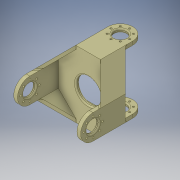
# Autodesk Inventor part: Coaxa 3 Machining
Saved by Autodesk Inventor 2016 (Build 200138000, 138)
## iProperties
Created: 2016-05-19
Part Number: Coaxa 3 Machining
Material: PET Plastic
Document SubType Name: Modeling
Designer: kromm.je.s
Density: 1.541 g/cm^3
Appearance: Smooth - Ash
Mass: 22.5167 g
Surface Area: 110.836 cm^2
Volume: 14.6118 cm^3
Author: kromm.je.s
Autodesk Inventor part; units mm, degrees
ref_plane "YZ Plane" through (0, 0, 0) normal (1, 0, 0) x (0, 1, 0)
sketch "Sketch1" plane through (0, 0, 0) normal (0, 0, 1) x (1, 0, 0)
  circle A0 centre (0, 0) radius 5
  circle A1 centre (0, 0) radius 10
  line L0 (0, 0) -> (-23, 0)
  line L1 (-23, 0) -> (-23, 27)
  line L2 (-23, 0) -> (-23, -27)
  line L3 (0, -10) -> (-23, -10)
  line L4 (0, 10) -> (-23, 10)
  line L5 (-23, 27) -> (-26, 27)
  line L6 (-26, 27) -> (-26, -27)
  line L7 (-26, -27) -> (-23, -27)
  dimension "d0" = 10
  dimension "d1" = 20
  dimension "d2" = 23
  dimension "d3" = 27
  dimension "d4" = 27
  dimension "d5" = 3
  constraints: 16 end point, 4 perpendicular, 3 point on line, 2 centre point, 2 coincident, 2 point on circle, 1 horizontal, 1 parallel, 1 tangent, 1 vertical
  measures "d0" diameter of A0
  measures "d1" diameter of A1
  measures "d2" distance of L0.start L0.end
  measures "d3" distance of L0.end L1.end
  measures "d4" distance of L0.end L2.end
  measures "d5" distance of L1.end L5.end
extrude "Extrusion1" add sketch "Sketch1" along normal blind 54
sketch "Sketch2" plane through (-23, 10, 0) normal (0, 1, 0) x (1, 0, 0)
  line L0 (0, 0) -> (-3, 0) projected
  line L1 (-3, 0) -> (-3, -54) projected
  line L2 (0, -54) -> (-3, -54) projected
  line L3 (0, 0) -> (0, -54) projected
  line L4 (23, 0) -> (0, 0) projected
  line L5 (0, -54) -> (0, 0) projected
  line L6 (23, -54) -> (0, -54) projected
  line L7 (23, 0) -> (23, -54) projected
  line L8 (23, 0) -> (23, -54) projected
  line L9 (23, -54) -> (23, -54) projected
  line L10 (23, 0) -> (23, -54) projected
  line L11 (23, 0) -> (23, 0) projected
  line L12 (0, 0) -> (23, 0) projected
  line L13 (0, 0) -> (0, -3)
  line L14 (0, -54) -> (0, -51)
  line L15 (0, 0) -> (0, -54) projected
  line L16 (33, 0) -> (33, -54) projected
  line L17 (0, -51) -> (33, -51)
  line L18 (33, -51) -> (33, -3)
  line L19 (33, -3) -> (0, -3)
  line L20 (0, -3) -> (0, -51)
  dimension "d8" = 3
  dimension "d9" = 3
  constraints: 12 end point, 3 point on line, 2 parallel, 1 horizontal, 1 perpendicular
  measures "d8" distance of L0.start L13.end
  measures "d9" distance of L5.start L14.end
extrude "Extrusion2" cut sketch "Sketch2" against normal blind 48 contours L19 L7 L17 L3 | L19 L16 L17 L7
sketch "Sketch3" plane through (-26, 27, 0) normal (0, 1, 0) x (1, 0, 0)
  line L0 (3, 0) -> (0, 0) projected
  line L1 (0, 0) -> (0, -54) projected
  line L2 (3, -54) -> (0, -54) projected
  line L3 (3, 0) -> (3, -54) projected
  line L4 (0, 0) -> (0, -54) projected
  line L5 (0, -27) -> (-23, -27)
  circle A0 centre (-23, -27) radius 5
  circle A1 centre (-23, -27) radius 10
  line L6 (-23, -17) -> (0, -17)
  line L7 (-23, -37) -> (0, -37)
  point P0 (26, 0)
  dimension "d12" = 23
  dimension "d13" = 10
  dimension "d14" = 20
  constraints: 6 end point, 2 centre point, 2 coincident, 2 perpendicular, 2 point on circle, 2 point on line, 1 horizontal, 1 midpoint, 1 tangent
  measures "d12" distance of L5.start L5.end
  measures "d13" diameter of A0
  measures "d14" diameter of A1
extrude "Extrusion3" add sketch "Sketch3" against normal blind 54 contours L1 L5 A1 L6 | L1 L7 A1 L5 | A1
sketch "Sketch4" plane through (0, 0, 0) normal (0, 0, -1) x (-1, 0, 0)
  line L0 (26, 27) -> (49, 27) projected
  line L1 (26, -27) -> (26, 27) projected
  line L2 (49, -27) -> (26, -27) projected
  line L3 (49, 27) -> (49, -27) projected
  line L4 (26, 27) -> (26, 24)
  line L5 (26, -27) -> (26, -24)
  line L6 (26, -27) -> (26, 27) projected
  line L7 (59, 27) -> (59, -27) projected
  line L8 (26, 21) -> (26, -24)
  line L9 (26, 24) -> (59, 24)
  line L10 (59, 24) -> (59, -24)
  line L11 (59, -24) -> (26, -24)
  line L12 (26, -24) -> (26, 24)
  point P0 (0, 0)
  dimension "d17" = 3
  dimension "d18" = 3
  constraints: 14 end point, 3 point on line, 2 parallel, 1 horizontal, 1 perpendicular
  measures "d17" distance of L0.start L4.end
  measures "d18" distance of L1.start L5.end
extrude "Extrusion4" cut sketch "Sketch4" against normal blind 48 contours L9 L3 L11 L1 | L9 L7 L11 L3
sketch "Sketch5" plane through (-26, -27, 54) normal (-1, 0, 0) x (0, 0, 1)
  line L0 (0, 54) -> (0, 0) projected
  line L1 (-17, 54) -> (0, 54) projected
  line L2 (-17, 3) -> (-17, 0) projected
  line L3 (-37, 51) -> (-37, 54) projected
  line L4 (-54, 54) -> (-37, 54) projected
  line L5 (-54, 54) -> (-54, 0) projected
  line L6 (-54, 0) -> (-37, 0) projected
  line L7 (-3, 17) -> (0, 17) projected
  line L8 (-3, 17) -> (0, 17) projected
  line L9 (0, 37) -> (-3, 37) projected
  line L10 (-3, 37) -> (0, 37) projected
  line L11 (-54, 37) -> (-51, 37) projected
  line L12 (-51, 37) -> (-54, 37) projected
  line L13 (-54, 17) -> (-51, 17) projected
  line L14 (-54, 17) -> (-51, 17) projected
  line L15 (-54, 17) -> (-51, 17) projected
  line L16 (-37, 0) -> (-54, 17)
  line L17 (-54, 54) -> (-37, 54) projected
  line L18 (-54, 37) -> (-37, 54)
  line L19 (0, 37) -> (-17, 54)
  line L20 (-17, 0) -> (0, 0) projected
  line L21 (-17, 0) -> (0, 17)
  line L22 (0, 0) -> (0, 17) projected
  line L23 (0, 54) -> (0, 0) projected
  line L24 (0, 17) -> (0, 0)
  line L25 (-17, 3) -> (-17, 0) projected
  line L26 (0, 0) -> (-17, 0)
  line L27 (-54, 0) -> (-37, 0) projected
  line L28 (-37, 0) -> (-54, 0)
  line L29 (-54, 0) -> (-54, 17) projected
  line L30 (-54, 0) -> (-54, 17)
  line L31 (-54, 37) -> (-54, 54)
  line L32 (-54, 54) -> (-37, 54)
  line L33 (0, 40) -> (0, 54)
  line L34 (0, 54) -> (-17, 54)
  line L35 (-54, 54) -> (0, 54) projected
  line L36 (-17, 0) -> (0, 0) projected
  line L37 (-37, 0) -> (-37, 3) projected
  line L38 (-37, 3) -> (-17, 3) projected
  line L39 (-17, 54) -> (-17, 51) projected
  line L40 (-37, 51) -> (-17, 51) projected
  point P0 (-54, 27)
  constraints: 24 end point, 4 collinear, 2 vertical, 1 horizontal, 1 perpendicular
extrude "Extrusion5" cut sketch "Sketch5" against normal blind 48 contours L0 L19 L1 | L18 L5 L4 | L0 L20 L21 | L16 L6 L5
sketch "Sketch6" plane through (-23, 27, 37) normal (1, 0, 0) x (0, 0, -1)
  line L0 (37, -17) -> (20, 0) projected
  line L1 (20, 0) -> (0, 0) projected
  line L2 (0, 0) -> (-17, -17) projected
  line L3 (-14, -17) -> (-14, -37) projected
  line L4 (-17, -37) -> (0, -54) projected
  line L5 (20, -54) -> (0, -54) projected
  line L6 (20, -54) -> (37, -37) projected
  line L7 (34, -17) -> (34, -37) projected
  line L8 (20, 0) -> (0, 0) projected
  line L9 (10, 0) -> (10, -54)
  circle A0 centre (10, -27) radius 10
  line L10 (-17, -17) -> (-14, -17) projected
  line L11 (-14, -37) -> (-17, -37) projected
  line L12 (37, -37) -> (34, -37) projected
  line L13 (34, -17) -> (37, -17) projected
  point P0 (37, -27)
  dimension "d26" = 20
  constraints: 3 midpoint, 2 end point, 1 centre point
  measures "d26" diameter of A0
extrude "Extrusion6" cut sketch "Sketch6" against normal blind 48 contours A0 L9 | L9 A0
sketch "Sketch7" plane through (-49, -27, 27) normal (0, -1, 0) x (1, 0, 0)
  circle A0 centre (0, 0) radius 7.5
  circle A1 centre (-7.5, 0) radius 0.75
  point P0 (49, -27)
  dimension "d32" = 15
  dimension "d33" = 1.5
  constraints: 1 centre point, 1 horizontal alignment, 2 other
  measures "d33" diameter of A1
extrude "Extrusion7" cut sketch "Sketch7" against normal blind 56 contours A1 A0 | A0 A1 picked at (-7.2472, 0) picked at (-7.7453, 0.0311)
pattern_circular "Circular Pattern1" count 8 over 360 about axis through (-49, 27, 27) along (0, -1, 0) of "Extrusion7"
sketch "Sketch8" plane through (0, 0, 0) normal (0, 0, -1) x (-1, 0, 0)
  circle A0 centre (0, 0) radius 7.5
  circle A1 centre (-7.5, 0) radius 0.75
  dimension "d39" = 15
  dimension "d40" = 1.5
  constraints: 1 centre point, 1 coincident, 1 horizontal alignment, 2 other
  measures "d40" diameter of A1
extrude "Extrusion8" cut sketch "Sketch8" against normal blind 56 contours A1 A0 | A0 A1 picked at (-7.2472, 0) picked at (-7.7453, 0.0311)
pattern_circular "Circular Pattern2" count 8 over 360 about axis through (0, 0, 0) along (0, 0, 1) of "Extrusion8"
chamfer "Chamfer3" [suppressed]
chamfer "Chamfer4" [suppressed]
sketch "Sketch9" plane through (-26, -10, 0) normal (-1, 0, 0) x (0, 0, 1)
  circle A0 centre (27, 10) radius 10 projected
  line L0 (0, 20) -> (17, 37) projected
  line L1 (17, 37) -> (37, 37) projected
  line L2 (37, 37) -> (54, 20) projected
  line L3 (54, 0) -> (37, -17) projected
  line L4 (17, -17) -> (37, -17) projected
  line L5 (17, -17) -> (0, 0) projected
  line L6 (54, 0) -> (37, -17) projected
  line L7 (37, -17) -> (37, -14)
  line L8 (37, -14) -> (40, -14)
  line L9 (37, -17) -> (40, -14)
  line L10 (17, -17) -> (17, -14)
  line L11 (17, -14) -> (14, -14)
  line L12 (14, -14) -> (17, -17)
  line L13 (0, 20) -> (17, 37) projected
  line L14 (17, 37) -> (17, 34)
  line L15 (17, 34) -> (14, 34)
  line L16 (14, 34) -> (17, 37)
  line L17 (17, 37) -> (37, 37) projected
  line L18 (37, 37) -> (54, 20) projected
  line L19 (37, 37) -> (37, 34)
  line L20 (37, 34) -> (40, 34)
  line L21 (40, 34) -> (37, 37)
  line L22 (54, 20) -> (51, 20) projected
  line L23 (51, 20) -> (51, 0) projected
  line L24 (51, 0) -> (54, 0) projected
  line L25 (0, 0) -> (3, 0) projected
  line L26 (3, 20) -> (3, 0) projected
  line L27 (3, 20) -> (0, 20) projected
  point P0 (0, 10)
  point P1 (7.99, 27.99)
  point P2 (46.01, 27.99)
  point P3 (46.01, -7.99)
  dimension "d52" = 3
  dimension "d53" = 3
  dimension "d54" = 3
  dimension "d55" = 3
  dimension "d56" = 3
  dimension "d57" = 3
  constraints: 24 end point, 16 point on line, 2 perpendicular, 2 vertical, 1 collinear
  measures "d52" distance of L3.end L7.end
  measures "d53" distance of L4.start L10.end
  measures "d54" distance of L10.end L11.end
  measures "d55" distance of L14.start L14.end
  measures "d56" distance of L14.end L15.end
  measures "d57" distance of L1.end L19.end
extrude "Extrusion9" [suppressed]
chamfer "Chamfer5" [suppressed]
sketch "Sketch10" plane through (-23, 27, 37) normal (1, 0, 0) x (0, 0, -1)
  circle A0 centre (10, -27) radius 10 projected
  line L0 (20, 0) -> (37, -17) projected
  line L1 (37, -17) -> (37, -37) projected
  line L2 (37, -37) -> (20, -54) projected
  line L3 (0, -54) -> (-17, -37) projected
  line L4 (-17, -17) -> (-17, -37) projected
  line L5 (-17, -17) -> (0, 0) projected
  line L6 (37, -37) -> (34, -37)
  line L7 (34, -37) -> (34, -40)
  line L8 (34, -40) -> (37, -37)
  line L9 (37, -37) -> (20, -54) projected
  line L10 (37, -17) -> (34, -17)
  line L11 (34, -17) -> (34, -14)
  line L12 (20, 0) -> (37, -17) projected
  line L13 (34, -14) -> (37, -17)
  line L14 (-17, -17) -> (-14, -17)
  line L15 (-14, -17) -> (-14, -14)
  line L16 (-14, -14) -> (-17, -17)
  line L17 (-17, -37) -> (-14, -37)
  line L18 (-14, -37) -> (-14, -40)
  line L19 (-14, -40) -> (-17, -37)
  line L20 (0, -51) -> (0, -54) projected
  line L21 (20, -54) -> (20, -51) projected
  line L22 (20, -51) -> (0, -51) projected
  line L23 (0, 0) -> (0, -3) projected
  line L24 (20, -3) -> (0, -3) projected
  line L25 (20, -3) -> (20, 0) projected
  point P0 (37, -27)
  point P1 (27.99, -7.99)
  point P2 (27.99, -46.01)
  dimension "d63" = 3
  dimension "d64" = 3
  dimension "d65" = 3
  dimension "d66" = 3
  dimension "d67" = 3
  dimension "d68" = 3
  dimension "d69" = 3
  dimension "d70" = 3
  constraints: 24 end point, 9 point on line, 2 horizontal, 1 perpendicular
  measures "d63" distance of L1.end L6.end
  measures "d64" distance of L6.end L7.end
  measures "d65" distance of L0.end L10.end
  measures "d66" distance of L10.end L11.end
  measures "d67" distance of L14.start L14.end
  measures "d68" distance of L14.end L15.end
  measures "d69" distance of L3.end L17.end
  measures "d70" distance of L17.end L18.end
extrude "Extrusion10" [suppressed]
chamfer "Chamfer6" [suppressed]
chamfer "Chamfer7" [suppressed]
fillet "Fillet1" [suppressed]
sketch "Sketch11" plane through (-23, -10, 51) normal (1, 0, 0) x (0, 0, -1)
  circle A0 centre (24, 10) radius 10 projected
  line L0 (51, 20) -> (34, 37) projected
  line L1 (34, 37) -> (14, 37) projected
  line L2 (14, 37) -> (-3, 20) projected
  line L3 (-3, 20) -> (0, 20) projected
  line L4 (0, 20) -> (0, 0) projected
  line L5 (0, 0) -> (-3, 0) projected
  line L6 (-3, 0) -> (14, -17) projected
  line L7 (34, -17) -> (14, -17) projected
  line L8 (34, -17) -> (51, 0) projected
  line L9 (51, 0) -> (48, 0) projected
  line L10 (48, 20) -> (48, 0) projected
  line L11 (48, 20) -> (51, 20) projected
  line L12 (14, 37) -> (14, 34)
  line L13 (34, 37) -> (14, 37) projected
  line L14 (34, 37) -> (34, 34)
  line L15 (34, 34) -> (48, 20)
  line L16 (34, 34) -> (14, 34) projected
  line L17 (-3, 20) -> (0, 20) projected
  line L18 (14, 34) -> (0, 20)
  line L19 (34, -17) -> (14, -17) projected
  line L20 (14, -14) -> (14, -17) projected
  line L21 (14, -17) -> (14, -14)
  line L22 (0, 0) -> (-3, 0) projected
  line L23 (14, -14) -> (0, 0)
  line L24 (34, -17) -> (34, -14)
  line L25 (34, -14) -> (48, 0)
  point P0 (51, 10)
  dimension "d82" = 3
  dimension "d83" = 3
  constraints: 16 end point, 3 vertical, 1 perpendicular
  measures "d82" distance of L6.end L20.start
  measures "d83" distance of L7.start L24.end
ref_plane "Work Plane5" through (-23, -27, 37) normal (0.7071068, 0, -0.7071068) x (0, 1, 0)
extrude "Extrusion11" add sketch "Sketch11" along normal up to surface contours L12 L18 L3 L2 | L23 L20 L6 L5 surface through (-23, -27, 37) normal (0.7071068, 0, -0.7071068)
ref_plane "Work Plane2" through (-23, -27, 17) normal (-0.7071068, 0, -0.7071068) x (0, 1, 0)
extrude "Extrusion12" add sketch "Sketch11" against normal up to surface contours L11 L15 L14 L0 | L9 L8 L24 L25 surface through (-23, -27, 17) normal (-0.7071068, 0, -0.7071068)
sketch "Sketch13" plane through (-26, -24, 17) normal (-1, 0, 0) x (0, 0, 1)
  circle A0 centre (10, 24) radius 10 projected
  line L0 (0, 51) -> (-17, 34) projected
  line L1 (-17, 34) -> (-17, 14) projected
  line L2 (-17, 14) -> (0, -3) projected
  line L3 (0, -3) -> (0, 0) projected
  line L4 (0, 0) -> (20, 0) projected
  line L5 (20, 0) -> (20, -3) projected
  line L6 (20, -3) -> (37, 14) projected
  line L7 (37, 34) -> (37, 14) projected
  line L8 (37, 34) -> (20, 51) projected
  line L9 (20, 51) -> (20, 48) projected
  line L10 (0, 48) -> (20, 48) projected
  line L11 (0, 48) -> (0, 51) projected
  line L12 (0, 51) -> (-17, 34) projected
  line L13 (-17, 34) -> (-14, 34)
  line L14 (-17, 14) -> (-14, 14)
  line L15 (34, 14) -> (37, 14) projected
  line L16 (37, 14) -> (34, 14)
  line L17 (34, 34) -> (37, 34) projected
  line L18 (37, 34) -> (34, 34)
  line L19 (34, 34) -> (20, 48)
  line L20 (-17, 34) -> (-14, 34) projected
  line L21 (0, 48) -> (20, 48) projected
  line L22 (-14, 34) -> (0, 48)
  line L23 (-14, 34) -> (0, 48) projected
  line L24 (-17, 14) -> (-14, 14) projected
  line L25 (-14, 14) -> (0, 0) projected
  line L26 (-14, 14) -> (0, 0)
  line L27 (34, 14) -> (20, 0) projected
  line L28 (34, 14) -> (20, 0)
  point P0 (-17, 24)
  dimension "d92" = 3
  dimension "d93" = 3
  dimension "d94" = 3
  dimension "d95" = 3
  constraints: 16 end point, 5 collinear, 2 horizontal
  measures "d92" distance of L0.end L13.end
  measures "d93" distance of L1.end L14.end
  measures "d94" distance of L6.end L15.start
  measures "d95" distance of L7.start L17.start
ref_plane "Work Plane3" through (-26, 10, 0) normal (-0.7071068, -0.7071068, 0) x (0, 0, 1)
ref_plane "Work Plane4" through (-26, -10, 0) normal (0.7071068, -0.7071068, 0) x (0, 0, 1)
extrude "Extrusion13" add sketch "Sketch13" against normal up to surface contours L11 L22 L13 L0 | L9 L8 L17 L19 surface through (-26, 10, 0) normal (-0.7071068, -0.7071068, 0)
extrude "Extrusion14" add sketch "Sketch13" along normal up to surface contours L14 L25 L3 L2 | L27 L15 L6 L5 surface through (-26, -10, 0) normal (0.7071068, -0.7071068, 0)
fillet "Fillet2" radius 1 8 edges at (-41.5, 25.5, 37) (-41.5, 25.5, 17) (-41.5, -25.5, 17) (-41.5, -25.5, 37) (-7.5, -10, 1.5) (-7.5, 10, 1.5) (-7.5, -10, 52.5) (-7.5, 10, 52.5)
fillet "Fillet4" radius 1 8 edges at (-26, -10, 52.5) (-26, 10, 52.5) (-26, -10, 1.5) (-26, 10, 1.5) (-23, 25.5, 17) (-23, -25.5, 17) (-23, -25.5, 37) (-23, 25.5, 37)
fillet "Fillet5" radius 1 8 edges at (-5, 0, 3) (-5, 0, 0) (-5, 0, 54) (-5, 0, 51) (-54, -24, 27) (-54, -27, 27) (-54, 27, 27) (-54, 24, 27)
fillet "Fillet6" radius 1 2 edges at (-26, 0, 37) (-23, 0, 37)
body "Solid1"
